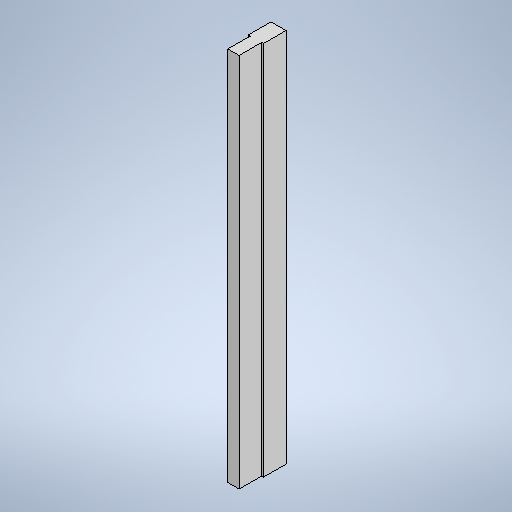
# Autodesk Inventor part: TRM 031 brush
Saved by Autodesk Inventor 2025.1 (Build 291241020, 241B)
## iProperties
Created: 2024-09-08
Part Number: TRM 031 brush
Material: Generic
Document SubType Name: Modeling
Designer: admin
Density: 1 g/cm^3
Appearance: Default
Author: admin
Autodesk Inventor part; units mm, degrees
ref_plane "YZ Plane" through (0, 0, 0) normal (1, 0, 0) x (0, 1, 0)
ref_plane "XZ Plane" through (0, 0, 0) normal (0, 1, 0) x (-1, 0, 0)
ref_plane "XY Plane" through (0, 0, 0) normal (0, 0, 1) x (1, 0, 0)
sketch "Sketch1" plane through (0, 0, 0) normal (0, 0, 1) x (1, 0, 0)
  line L0 (-10, 0) -> (10, 0)
  line L1 (10, 0) -> (10, -30)
  line L2 (10, -30) -> (-10, -30)
  line L3 (-10, -30) -> (-10, 0)
  line L4 (7.5, -30) -> (-7.5, -30)
  line L5 (-7.5, -30) -> (-7.5, -60)
  line L6 (-7.5, -60) -> (7.5, -60)
  line L7 (7.5, -60) -> (7.5, -30)
  point P0 (0, 0)
  point P1 (0, 0)
  point P2 (0, -30)
  dimension "d0" = 20
  dimension "d1" = 30
  dimension "d2" = 15
  dimension "d3" = 30
  constraints: 16 end point, 4 parallel, 3 midpoint, 2 horizontal, 2 perpendicular, 1 coincident, 1 point on line
  measures "d0" distance of L0.start L0.end
  measures "d1" distance of L0.end L1.end
  measures "d2" distance of L5.end L6.end
  measures "d3" distance of L6.end L4.start
extrude "Extrusion1" add sketch "Sketch1" along normal blind 500
equation "\"d3\" = d1"
body "Solid1"
